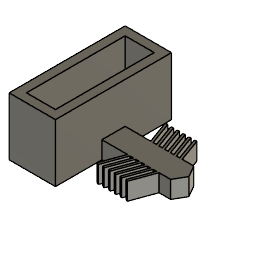
DRAFT-UNTESTED Zip-tie push-in clip (Autodesk Fusion 360 design; units mm, degrees)
Autodesk Fusion 360 part; units mm, degrees
sketch "Sketch1" plane through (0, 0, 0) normal (0, 0, 1) x (1, 0, 0)
  line L0 (0, 0) -> (-24.511, 0)
  line L1 (0, 0) -> (-1.1547, 2)
  line L2 (-1.1547, 2) -> (-3.1547, 2)
  line L3 (-3.1547, 2) -> (-4.6106, 6)
  line L4 (-4.6106, 6) -> (-4.9865, 5.8632)
  line L5 (-4.9865, 5.8632) -> (-3.5804, 2)
  line L6 (-3.5804, 2) -> (-4.1547, 2)
  line L7 (-4.5804, 2) -> (-5.1547, 2)
  line L8 (-5.9865, 5.8632) -> (-4.5804, 2)
  line L9 (-5.6106, 6) -> (-5.9865, 5.8632)
  line L10 (-4.1547, 2) -> (-5.6106, 6)
  line L11 (-5.5804, 2) -> (-6.1547, 2)
  line L12 (-6.9865, 5.8632) -> (-5.5804, 2)
  line L13 (-6.6106, 6) -> (-6.9865, 5.8632)
  line L14 (-5.1547, 2) -> (-6.6106, 6)
  line L15 (-6.5804, 2) -> (-7.1547, 2)
  line L16 (-7.9865, 5.8632) -> (-6.5804, 2)
  line L17 (-7.6106, 6) -> (-7.9865, 5.8632)
  line L18 (-6.1547, 2) -> (-7.6106, 6)
  line L19 (-7.5804, 2) -> (-8.1547, 2)
  line L20 (-8.9865, 5.8632) -> (-7.5804, 2)
  line L21 (-8.6106, 6) -> (-8.9865, 5.8632)
  line L22 (-7.1547, 2) -> (-8.6106, 6)
  line L23 (-8.5804, 2) -> (-9.1547, 2)
  line L24 (-9.9865, 5.8632) -> (-8.5804, 2)
  line L25 (-9.6106, 6) -> (-9.9865, 5.8632)
  line L26 (-8.1547, 2) -> (-9.6106, 6)
  line L27 (-9.1547, 2) -> (-12.9865, 2)
  line L28 (-20.9865, 10) -> (-20.9865, 0)
  line L29 (-12.9865, 2) -> (-12.9865, 10)
  line L30 (-12.9865, 10) -> (-20.9865, 10)
  line L31 (-12.9865, 2) -> (-12.9865, 0)
  line L32 (-9.6106, -6) -> (-9.9865, -5.8632)
  line L33 (-9.9865, -5.8632) -> (-8.5804, -2)
  line L34 (-7.1547, -2) -> (-8.6106, -6)
  line L35 (-5.1547, -2) -> (-6.6106, -6)
  line L36 (-9.1547, -2) -> (-12.9865, -2)
  line L37 (-7.5804, -2) -> (-8.1547, -2)
  line L38 (-3.5804, -2) -> (-4.1547, -2)
  line L39 (-20.9865, -10) -> (-20.9865, 0)
  line L40 (-12.9865, -10) -> (-20.9865, -10)
  line L41 (0, 0) -> (-1.1547, -2)
  line L42 (-4.9865, -5.8632) -> (-3.5804, -2)
  line L43 (-5.6106, -6) -> (-5.9865, -5.8632)
  line L44 (-6.5804, -2) -> (-7.1547, -2)
  line L45 (-7.6106, -6) -> (-7.9865, -5.8632)
  line L46 (-12.9865, -2) -> (-12.9865, -10)
  line L47 (-8.5804, -2) -> (-9.1547, -2)
  line L48 (-6.6106, -6) -> (-6.9865, -5.8632)
  line L49 (-12.9865, -2) -> (-12.9865, 0)
  line L50 (-7.9865, -5.8632) -> (-6.5804, -2)
  line L51 (-8.6106, -6) -> (-8.9865, -5.8632)
  line L52 (-6.1547, -2) -> (-7.6106, -6)
  line L53 (-4.6106, -6) -> (-4.9865, -5.8632)
  line L54 (-3.1547, -2) -> (-4.6106, -6)
  line L55 (-8.9865, -5.8632) -> (-7.5804, -2)
  line L56 (-8.1547, -2) -> (-9.6106, -6)
  line L57 (-6.9865, -5.8632) -> (-5.5804, -2)
  line L58 (-4.1547, -2) -> (-5.6106, -6)
  line L59 (-1.1547, -2) -> (-3.1547, -2)
  line L60 (-5.9865, -5.8632) -> (-4.5804, -2)
  line L61 (-4.5804, -2) -> (-5.1547, -2)
  line L62 (-5.5804, -2) -> (-6.1547, -2)
  line L63 (-14.4865, 2) -> (-14.4865, 0)
  line L64 (-14.4865, -2) -> (-14.4865, 0)
  line L65 (-14.4865, -2) -> (-14.4865, -8.5)
  line L66 (-14.4865, -8.5) -> (-19.4865, -8.5)
  line L67 (-19.4865, -8.5) -> (-19.4865, 0)
  line L68 (-19.4865, 8.5) -> (-19.4865, 0)
  line L69 (-14.4865, 8.5) -> (-19.4865, 8.5)
  line L70 (-14.4865, 2) -> (-14.4865, 8.5)
  point P0 (-24.511, 0)
  dimension "d1" = 4
  dimension "d2" = 0.4
  dimension "d3" = 1
  dimension "d6" = -1
  dimension "d7" = 0
  dimension "d8" = 110
  dimension "d9" = 4
  dimension "d10" = 8
  dimension "d11" = 8
  dimension "d12" = 3
  dimension "d13" = 2
  dimension "d14" = 60
  dimension "d19" = 1.5
  constraint coincident L0.start L1.start
  constraint horizontal L0
  constraint coincident L0 L1.start
  constraint horizontal L2
  constraint perpendicular L3 L4
  constraint perpendicular L4 L5
  constraint horizontal L6
  constraint coincident L19.end L26.start
  constraint parallel L23 L27
  constraint coincident L0 L28.end
  constraint perpendicular L0 L28
  constraint perpendicular L27 L29
  constraint horizontal L30
  constraint coincident L0 L31.end
  constraint perpendicular L0 L31
  constraint symmetric L1.start L0 L41.start
  constraint symmetric P0 L0 L0.end
  constraint symmetric L0 L1.start L41.start
  constraint symmetric L0 L1.end L41.end
  constraint symmetric L0 L2.end L54.start
  constraint symmetric L0 L3.end L53.start
  constraint symmetric L0 L4.end L42.start
  constraint symmetric L0 L5.end L38.start
  constraint symmetric L0 L6.end L38.end
  constraint symmetric L0 L7.start L60.end
  constraint symmetric L0 L7.end L35.start
  constraint symmetric L0 L8.start L43.end
  constraint symmetric L0 L9.start L43.start
  constraint symmetric L0 L11.start L57.end
  constraint symmetric L0 L11.end L52.start
  constraint symmetric L0 L12.start L48.end
  constraint symmetric L0 L13.start L35.end
  constraint symmetric L0 L15.start L44.start
  constraint symmetric L0 L15.end L34.start
  constraint symmetric L0 L16.start L45.end
  constraint symmetric L0 L17.start L45.start
  constraint symmetric L0 L19.start L37.start
  constraint symmetric L0 L19.end L37.end
  constraint symmetric L0 L20.start L51.end
  constraint symmetric L0 L21.start L34.end
  constraint symmetric L0 L23.start L33.end
  constraint symmetric L0 L23.end L36.start
  constraint symmetric L0 L24.start L32.end
  constraint symmetric L0 L25.start L32.start
  constraint symmetric L0 L27.end L36.end
  constraint symmetric L0 L28.start L39.start
  constraint symmetric L0 L28.end L39.end
  constraint symmetric L0 L29.end L40.start
  constraint symmetric L0 L31.end L49.end
  measures "d2" distance of L3 L5
  measures "d3" distance of L2.end L6.end
  measures "d8" angle of L19 L26
  measures "d9" distance of L23 L25.start
  measures "d10" distance of L27.end L29.end
  measures "d11" distance of L28.start L29.end
  measures "d12" distance of L24.start L29
  measures "d13" distance of L1.end L2.end
  measures "d14" angle of L0 L1
extrude "Extrude1" add sketch "Sketch1" along normal blind 3 contours L0 L32 L33 L34 L35 L36 L37 L38 L41 L42 L43 L44 L45 L47 L48 L49 L50 L51 L52 L53 L54 L55 L56 L57 L58 L59 L60 L61 L62 | L0 L1 L2 L3 L4 L5 L6 L7 L8 L9 L10 L11 L12 L13 L14 L15 L16 L17 L18 L19 L20 L21 L22 L23 L24 L25 L26 L27 L31
extrude "Extrude2" add sketch "Sketch1" along normal blind 10 contours L0 L39 L40 L46 L49 L64 L65 L66 L67 | L0 L28 L29 L30 L31 L63 L68 L69 L70
